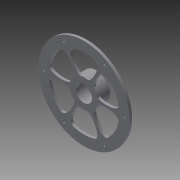
# Autodesk Inventor part: Hub_Carrier
Saved by Autodesk Inventor 2016 (Build 200138000, 138)
## iProperties
Created: 2015-06-04
Part Number: Hub_Carrier
Material: Generic
Document SubType Name: Modeling
Designer: Yann
Density: 1 g/cm^3
Appearance: Default
Author: Yann
Autodesk Inventor part; units mm, degrees
ref_plane "YZ Plane" through (0, 0, 0) normal (1, 0, 0) x (0, 1, 0)
sketch "Sketch1" plane through (0, 0, 0) normal (0, 1, 0) x (-1, 0, 0)
  line L0 (0, -39.2) -> (0, 39.2) construction
  line L1 (-39.2, 0) -> (39.2, 0) construction
  circle A0 centre (0, 0) radius 21 projected
  circle A1 centre (0, 0) radius 28
  circle A2 centre (-24.5, 0) radius 2
  circle A3 centre (12.25, -21.2176) radius 2
  circle A4 centre (12.25, 21.2176) radius 2
  point P0 (0, 0)
  dimension "d0" = 7
  dimension "d1" = 4
  dimension "d2" = 24.5
  dimension "d3" = 42
  dimension "d6" = 360
  constraints: 4 centre point, 1 coincident, 1 point on line, 7 other
  measures "d0" radial gap between concentric circles of A0 A1
  measures "d1" diameter of A2
  measures "d2" distance of A2.centre A1.centre
  measures "d3" diameter of A0
ref_plane "Work Plane1" through (-25.1666, 9.5, -25.1666) normal (0, 1, 0) x (-0.3064381, 0, 0.9518906)
ref_plane "Work Plane2" through (-25.1666, -9.5, -25.1666) normal (0, -1, 0) x (0.9518906, 0, 0.3064381)
extrude "Extrusion1" add sketch "Sketch1" against normal up to surface (19 mm away) from surface at 9.5
sketch "Sketch2" plane through (0, -9.5, 0) normal (0, -1, 0) x (1, 0, 0)
  line L0 (0, 126) -> (0, -126) construction
  line L1 (-126, 0) -> (126, 0) construction
  circle A0 centre (0, 0) radius 21 construction
  circle A1 centre (0, 0) radius 16
  circle A2 centre (0, 0) radius 90
  circle A3 centre (0, 0) radius 70 construction
  circle A4 centre (80, 0) radius 2
  circle A5 centre (40, 69.282) radius 2
  circle A6 centre (-40, 69.282) radius 2
  circle A7 centre (-80, 0) radius 2
  circle A8 centre (-40, -69.282) radius 2
  circle A9 centre (40, -69.282) radius 2
  circle A10 centre (0, 0) radius 28 construction
  line L2 (68.6686, -13.5874) -> (70, 0) construction
  line L3 (70, 0) -> (27.9999, 0.0658) construction
  circle A11 centre (0, 0) radius 28 construction
  line L4 (27.9999, 0.0658) -> (26.9082, -7.7428) construction
  spline S0 degree 3 poles (68.6686, -13.5874) (70, 0) (27.9999, 0.0658) (26.9082, -7.7428) knots 1 1 1 1 2 2 2 2
  line L5 (68.6686, 13.5874) -> (70, 0) construction
  line L6 (70, 0) -> (27.9999, -0.0658) construction
  line L7 (27.9999, -0.0658) -> (26.9082, 7.7428) construction
  spline S1 degree 3 poles (68.6686, 13.5874) (70, 0) (27.9999, -0.0658) (26.9082, 7.7428) knots 1 1 1 1 2 2 2 2
  spline S2 degree 3 poles (46.1014, 52.6751) (35, 60.6218) (13.943, 24.2815) (20.1595, 19.4318) knots 1 1 1 1 2 2 2 2
  line L8 (46.1014, 52.6751) -> (35, 60.6218) construction
  line L9 (35, 60.6218) -> (13.943, 24.2815) construction
  line L10 (13.943, 24.2815) -> (20.1595, 19.4318) construction
  spline S3 degree 3 poles (22.5673, 66.2625) (35, 60.6218) (14.057, 24.2157) (6.7486, 27.1745) knots 1 1 1 1 2 2 2 2
  line L11 (22.5673, 66.2625) -> (35, 60.6218) construction
  line L12 (35, 60.6218) -> (14.057, 24.2157) construction
  line L13 (14.057, 24.2157) -> (6.7486, 27.1745) construction
  spline S4 degree 3 poles (-22.5673, 66.2625) (-35, 60.6218) (-14.057, 24.2157) (-6.7486, 27.1745) knots 1 1 1 1 2 2 2 2
  line L14 (-22.5673, 66.2625) -> (-35, 60.6218) construction
  line L15 (-35, 60.6218) -> (-14.057, 24.2157) construction
  line L16 (-14.057, 24.2157) -> (-6.7486, 27.1745) construction
  spline S5 degree 3 poles (-46.1014, 52.6751) (-35, 60.6218) (-13.943, 24.2815) (-20.1595, 19.4318) knots 1 1 1 1 2 2 2 2
  line L17 (-46.1014, 52.6751) -> (-35, 60.6218) construction
  line L18 (-35, 60.6218) -> (-13.943, 24.2815) construction
  line L19 (-13.943, 24.2815) -> (-20.1595, 19.4318) construction
  spline S6 degree 3 poles (-68.6686, 13.5874) (-70, 0) (-27.9999, -0.0658) (-26.9082, 7.7428) knots 1 1 1 1 2 2 2 2
  line L20 (-68.6686, 13.5874) -> (-70, 0) construction
  line L21 (-70, 0) -> (-27.9999, -0.0658) construction
  line L22 (-27.9999, -0.0658) -> (-26.9082, 7.7428) construction
  spline S7 degree 3 poles (-68.6686, -13.5874) (-70, 0) (-27.9999, 0.0658) (-26.9082, -7.7428) knots 1 1 1 1 2 2 2 2
  line L23 (-68.6686, -13.5874) -> (-70, 0) construction
  line L24 (-70, 0) -> (-27.9999, 0.0658) construction
  line L25 (-27.9999, 0.0658) -> (-26.9082, -7.7428) construction
  spline S8 degree 3 poles (-46.1014, -52.6751) (-35, -60.6218) (-13.943, -24.2815) (-20.1595, -19.4318) knots 1 1 1 1 2 2 2 2
  line L26 (-46.1014, -52.6751) -> (-35, -60.6218) construction
  line L27 (-35, -60.6218) -> (-13.943, -24.2815) construction
  line L28 (-13.943, -24.2815) -> (-20.1595, -19.4318) construction
  spline S9 degree 3 poles (-22.5673, -66.2625) (-35, -60.6218) (-14.057, -24.2157) (-6.7486, -27.1745) knots 1 1 1 1 2 2 2 2
  line L29 (-22.5673, -66.2625) -> (-35, -60.6218) construction
  line L30 (-35, -60.6218) -> (-14.057, -24.2157) construction
  line L31 (-14.057, -24.2157) -> (-6.7486, -27.1745) construction
  spline S10 degree 3 poles (22.5673, -66.2625) (35, -60.6218) (14.057, -24.2157) (6.7486, -27.1745) knots 1 1 1 1 2 2 2 2
  line L32 (22.5673, -66.2625) -> (35, -60.6218) construction
  line L33 (35, -60.6218) -> (14.057, -24.2157) construction
  line L34 (14.057, -24.2157) -> (6.7486, -27.1745) construction
  spline S11 degree 3 poles (46.1014, -52.6751) (35, -60.6218) (13.943, -24.2815) (20.1595, -19.4318) knots 1 1 1 1 2 2 2 2
  line L35 (46.1014, -52.6751) -> (35, -60.6218) construction
  line L36 (35, -60.6218) -> (13.943, -24.2815) construction
  line L37 (13.943, -24.2815) -> (20.1595, -19.4318) construction
  arc A12 (46.1014, -52.6751) -> (68.6686, -13.5874) centre (0, 0) ccw
  arc A13 (20.1595, -19.4318) -> (26.9082, -7.7428) centre (0, 0) ccw
  arc A14 (-22.5673, -66.2625) -> (22.5673, -66.2625) centre (0, 0) ccw
  arc A15 (-68.6686, -13.5874) -> (-46.1014, -52.6751) centre (0, 0) ccw
  arc A16 (-46.1014, 52.6751) -> (-68.6686, 13.5874) centre (0, 0) ccw
  arc A17 (22.5673, 66.2625) -> (-22.5673, 66.2625) centre (0, 0) ccw
  arc A18 (68.6686, 13.5874) -> (46.1014, 52.6751) centre (0, 0) ccw
  arc A19 (-26.9082, -7.7428) -> (-20.1595, -19.4318) centre (0, 0) ccw
  arc A20 (-20.1595, 19.4318) -> (-26.9082, 7.7428) centre (0, 0) ccw
  arc A21 (6.7486, 27.1745) -> (-6.7486, 27.1745) centre (0, 0) ccw
  arc A22 (26.9082, 7.7428) -> (20.1595, 19.4318) centre (0, 0) ccw
  arc A23 (-6.7486, -27.1745) -> (6.7486, -27.1745) centre (0, 0) ccw
  point P0 (0, 0)
  dimension "d10" = 5
  dimension "d11" = 180
  dimension "d12" = 20
  dimension "d13" = 4
  dimension "d14" = 80
  dimension "d17" = 360
  dimension "d21" = 360
  constraints: 30 point on circle, 21 centre point, 14 coincident, 3 symmetric about line, 1 point on line, 140 other
  measures "d10" radial gap between concentric circles of A0 A1
  measures "d11" diameter of A2
  measures "d12" radial gap between concentric circles of A2 A3
  measures "d13" diameter of A4
  measures "d14" distance of point (0, 0) A4.centre
extrude "Extrusion2" add sketch "Sketch2" along normal blind 5
equation "\"d2\" = 0.5 * d3 + 0.5 * d0"
equation "\"d14\" = 0.5 * d11 - 0.5 * d12"
body "Solid1"
